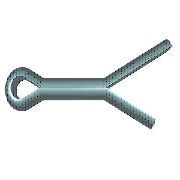
# Autodesk Inventor part: ISO 1234 - 2,5 x 12
Saved by Autodesk Inventor 2024.4 (Build 284460000, 460)
## iProperties
Created: 2023-01-19
Part Number: ISO 1234 - 2,5 x 12
Material: Stahl
Description: Splint
Document SubType Name: Modeling
Standard: ISO 1234
Designer: windows-desktop
Standard Revision: 1998
Standards Organization: DIN
Language: de-DE
Size Designation: 2,5 x 12
Categories: <MemberInstance><Categories><Category DisplayName="Verbindungselemente" InternalName="e4da775c-781d-43d5-af7c-5136215cf5a6" Mnemonic="FSTN"><Category DisplayName="Stifte" InternalName="3b3d1810-ac9b-4ede-8c7f-cc6b956350b0" Mnemonic="PIN"><CategoryParameter DisplayName="Nenndurchmesser" InternalName="6cc331d7-8ea1-4fca-9c9a-55ec966217e5" Mnemonic="nomdia"/><CategoryParameter DisplayName="Nennlänge" InternalName="897bd938-6adf-4e3c-a2d4-0d7cae45eecd" Mnemonic="nomlen"/><Category DisplayName="Splinte" InternalName="4383ab9c-662d-4701-a95a-d5834a9f0a34" Mnemonic="SPLTPIN"><CategoryParameter DisplayName="Bolzendurchmesser" InternalName="761c08f3-f58b-48c9-8a5c-1931069602db" Mnemonic="bltdia"/></Category></Category></Category><Category DisplayName="Datentyp" InternalName="23b78d0f-2648-40c6-8793-ca6db495c9e8" Mnemonic="DATATYPE"><CategoryParameter DisplayName="Anzeigename" InternalName="05415f3d-3907-474b-a020-eb9d644f4cf3" Mnemonic="DISPLAYNAME"/><CategoryParameter DisplayName="Norm" InternalName="0c0a119c-1e12-4c84-803f-101930972f5e" Mnemonic="STANDARD"/><CategoryParameter DisplayName="Beschreibung" InternalName="13903e3d-64b1-4950-80da-f627842ea37f" Mnemonic="DESCRIPTION"/><CategoryParameter DisplayName="Bezeichnung" InternalName="2675968c-4ce5-49e0-a4f5-552d29089031" Mnemonic="DESIGNATION"/><CategoryParameter DisplayName="Standardzeile" InternalName="2af9ec52-faaa-4026-b378-f9fa4afca842" Mnemonic="DEFAULTROW"/><CategoryParameter DisplayName="Ordnername" InternalName="3f06958e-8713-4116-9be7-ed6184ecc97b" Mnemonic="FOLDERNAME"/><CategoryParameter DisplayName="Revisionsanleitung" InternalName="45a75005-10b1-4dfc-8d6d-dfe629f0b93c" Mnemonic="REVISIONGUID"/><CategoryParameter DisplayName="Dateiname" InternalName="8b46a4cc-9585-4fed-90c3-899f57e09a73" Mnemonic="FILENAME"/><CategoryParameter DisplayName="Normungsorganisation" InternalName="8f5914e1-4693-403f-8ab5-d37768198c9d" Mnemonic="STDSORG"/><CategoryParameter DisplayName="Gruppenversion" InternalName="914462f6-6e19-4b14-ba84-155b9680b1d0" Mnemonic="FAMILYREVISION"/><CategoryParameter DisplayName="Normrevision" InternalName="91d5a463-65c2-4fde-b823-3b7fea5e8e17" Mnemonic="STANDARDREVISION"/><CategoryParameter DisplayName="Variantenrevision" InternalName="a65d44b9-392f-4f4f-857b-e4b3d54996fe" Mnemonic="MEMBERREVISION"/><CategoryParameter DisplayName="ClipFormat" InternalName="bc51e27b-3422-4e78-93ef-cec197ddf230" Mnemonic="CLIPFORMAT"/><CategoryParameter DisplayName="Hersteller" InternalName="cd6c7a72-a28a-4e50-99a9-2c7f4e13e5ad" Mnemonic="MANUFACTURER"/><CategoryParameter DisplayName="InternerName" InternalName="cf1d0246-76d9-4b4a-8305-fa0409afb5c1" Mnemonic="INTERNALNAME"/><CategoryParameter DisplayName="IstMetrisch" InternalName="e2385c5b-1ea4-4823-96a8-8de651266ec3" Mnemonic="ISMETRIC"/><Category DisplayName="Bauteil" InternalName="c0e0b642-3bcb-4cc8-9e80-f96d35c4afa4" Mnemonic="PART"><CategoryParameter DisplayName="Bauteilnummer" InternalName="016b6077-bfbe-49bd-92c9-d8d59c39c941" Mnemonic="PARTNUMBER"/><CategoryParameter DisplayName="Bestandsnummer" InternalName="4dba7c1c-e26c-444e-836c-b08b433409a8" Mnemonic="STOCKNUMBER"/><CategoryParameter DisplayName="Materialschlüssel" InternalName="5c9a8adb-dd2b-4535-b97f-0a94a95fe41f" Mnemonic="MATERIALKEY"/><CategoryParameter DisplayName="Material" InternalName="818a152a-d3c3-49ca-80ee-df7d91421b8e" Mnemonic="MATERIAL"/></Category></Category><Category DisplayName="ÄltereVersionenzuweisen" InternalName="cd87c42b-3e48-431e-b5c0-1cbeb14dfe77" Mnemonic="LEGACYMAP"><CategoryParameter DisplayName="Eindeutige DA-Varianten-ID" InternalName="0918ad47-427f-4fed-ae26-24c81c58f590" Mnemonic="DACOOKIE"/><CategoryParameter DisplayName="ID zusammenführen" InternalName="0ee8fb18-e2ed-4f39-96f6-1f4b5f50aa71" Mnemonic="MERGE11"/><CategoryParameter DisplayName="Eindeutige CC-Varianten-ID" InternalName="5193edd4-b2b0-4ab4-9d54-de900eee34e0" Mnemonic="CCCOOKIE"/><CategoryParameter DisplayName="ID aufteilen" InternalName="72b5c83c-be7f-45c4-ae51-9160ea6deb26" Mnemonic="SPLIT"/><CategoryParameter DisplayName="VarianteID" InternalName="8e5e0294-fc51-4c8f-b3d7-003dc5ed94f6" Mnemonic="MEMBERID"/><CategoryParameter DisplayName="Katalogname" InternalName="d99d1e27-aa94-4de2-af4c-c348882a6f4f" Mnemonic="CATALOGNAME"/><CategoryParameter DisplayName="Gruppennummer" InternalName="e705e1f4-09cb-413e-91f9-551b4188271e" Mnemonic="FAMILYNUMBER"/></Category></Categories><FamilyTemplate Id="si0028"><FamilyTemplateParameters><FamilyTemplateParameter ObjectType="kUserParameterObject" ValueType="xs:double" Id="1" ObjectReferenceKey="KBR"/><FamilyTemplateParameter ObjectType="kUserParameterObject" ValueType="xs:double" Id="2" ObjectReferenceKey="NNDMAX"/><FamilyTemplateParameter ObjectType="kUserParameterObject" ValueType="xs:double" Id="3" ObjectReferenceKey="DSH"/><FamilyTemplateParameter ObjectType="kUserParameterObject" ValueType="xs:double" Id="4" ObjectReferenceKey="MSIAB"/><FamilyTemplateParameter ObjectType="kUserParameterObject" ValueType="xs:double" Id="5" ObjectReferenceKey="SNLG"/><FamilyTemplateParameter ObjectType="kUserParameterObject" ValueType="xs:double" Id="6" ObjectReferenceKey="SNND"/><FamilyTemplateParameter ObjectType="kUserParameterObject" ValueType="xs:double" Id="7" ObjectReferenceKey="KOL"/><FamilyTemplateParameter ObjectType="kUserParameterObject" ValueType="xs:double" Id="8" ObjectReferenceKey="LGDIF"/><FamilyTemplateParameter ObjectType="kUserParameterObject" ValueType="xs:double" Id="9" ObjectReferenceKey="NNDMIN"/><FamilyTemplateParameter ObjectType="kUserParameterObject" ValueType="xs:double" Id="10" ObjectReferenceKey="SNND1"/><FamilyTemplateParameter ObjectType="kPropertyObject" ValueType="xs:string" Id="100" ObjectReferenceKey="{32853F0F-3444-11d1-9E93-0060B03C1CA6}" SubObjectId="52"/><FamilyTemplateParameter ObjectType="kPropertyObject" ValueType="xs:string" Id="105" ObjectReferenceKey="{32853F0F-3444-11d1-9E93-0060B03C1CA6}" SubObjectId="5"/><FamilyTemplateParameter ObjectType="kPartComponentDefinitionObject" ValueType="xs:string" Id="110" SubObjectId="Material"/></FamilyTemplateParameters></FamilyTemplate><CategoryParameterMap><ParamToTemplateMap><ParamToTemplate CategoryParameter="//CategoryParameter[@InternalName='05415f3d-3907-474b-a020-eb9d644f4cf3']" ConstantValue="DIN EN ISO 1234"/><ParamToTemplate CategoryParameter="//CategoryParameter[@InternalName='cf1d0246-76d9-4b4a-8305-fa0409afb5c1']" ConstantValue="e94eddc3-8f06-45e0-83a1-c6f48b028452"/><ParamToTemplate CategoryParameter="//CategoryParameter[@InternalName='3f06958e-8713-4116-9be7-ed6184ecc97b']" ConstantValue="ISO 1234(1)"/><ParamToTemplate CategoryParameter="//CategoryParameter[@InternalName='914462f6-6e19-4b14-ba84-155b9680b1d0']" ConstantValue="10"/><ParamToTemplate CategoryParameter="//CategoryParameter[@InternalName='bc51e27b-3422-4e78-93ef-cec197ddf230']" ConstantValue="CF_INVENTOR.STDPARTS"/><ParamToTemplate CategoryParameter="//CategoryParameter[@InternalName='e2385c5b-1ea4-4823-96a8-8de651266ec3']" ConstantValue="true"/><ParamToTemplate CategoryParameter="//CategoryParameter[@InternalName='13903e3d-64b1-4950-80da-f627842ea37f']" ConstantValue="Split Pin"/><ParamToTemplate CategoryParameter="//CategoryParameter[@InternalName='8f5914e1-4693-403f-8ab5-d37768198c9d']" ConstantValue="DIN"/><ParamToTemplate CategoryParameter="//CategoryParameter[@InternalName='0c0a119c-1e12-4c84-803f-101930972f5e']" ConstantValue="ISO 1234"/><ParamToTemplate CategoryParameter="//CategoryParameter[@InternalName='cd6c7a72-a28a-4e50-99a9-2c7f4e13e5ad']" TemplateParameter="104"/><ParamToTemplate CategoryParameter="//CategoryParameter[@InternalName='91d5a463-65c2-4fde-b823-3b7fea5e8e17']" ConstantValue="1998"/><ParamToTemplate CategoryParameter="//CategoryParameter[@InternalName='45a75005-10b1-4dfc-8d6d-dfe629f0b93c']" ConstantValue="dfdbe262-4242-467a-bd84-0a8edc805856"/><ParamToTemplate CategoryParameter="//CategoryParameter[@InternalName='2af9ec52-faaa-4026-b378-f9fa4afca842']" ConstantValue="10"/><ParamToTemplate CategoryParameter="//CategoryParameter[@InternalName='d99d1e27-aa94-4de2-af4c-c348882a6f4f']" ConstantValue="DIN"/><ParamToTemplate CategoryParameter="//CategoryParameter[@InternalName='e705e1f4-09cb-413e-91f9-551b4188271e']" ConstantValue="220"/><ParamToTemplate CategoryParameter="//CategoryParameter[@InternalName='8b46a4cc-9585-4fed-90c3-899f57e09a73']" ConstantValue="ISO 1234 - 2,5 x 12DIN EN"/><ParamToTemplate CategoryParameter="//CategoryParameter[@InternalName='a65d44b9-392f-4f4f-857b-e4b3d54996fe']" ConstantValue="35897454-1E07-4AEE-A925-0F5C18AD98F7"/><ParamToTemplate CategoryParameter="//CategoryParameter[@InternalName='8e5e0294-fc51-4c8f-b3d7-003dc5ed94f6']" ConstantValue="540"/><ParamToTemplate CategoryParameter="//CategoryParameter[@InternalName='2675968c-4ce5-49e0-a4f5-552d29089031']" TemplateParameter="100"/><ParamToTemplate CategoryParameter="//CategoryParameter[@InternalName='818a152a-d3c3-49ca-80ee-df7d91421b8e']" TemplateParameter="110"/><ParamToTemplate CategoryParameter="//CategoryParameter[@InternalName='761c08f3-f58b-48c9-8a5c-1931069602db']" TemplateParameter="2"/><ParamToTemplate CategoryParameter="//CategoryParameter[@InternalName='016b6077-bfbe-49bd-92c9-d8d59c39c941']" TemplateParameter="105"/><ParamToTemplate CategoryParameter="//CategoryParameter[@InternalName='897bd938-6adf-4e3c-a2d4-0d7cae45eecd']" TemplateParameter="5"/><ParamToTemplate CategoryParameter="//CategoryParameter[@InternalName='6cc331d7-8ea1-4fca-9c9a-55ec966217e5']" TemplateParameter="6"/></ParamToTemplateMap></CategoryParameterMap></MemberInstance>
Mass: 0.700909 g
Surface Area: 2.16494 cm^2
Volume: 0.0892877 cm^3
Density: 7.85 g/cm^3
Appearance: Platte
IsCustomPart: 0
Author: windows-desktop
Autodesk Inventor part; units mm, degrees
ref_plane "YZ Plane" through (0, 0, 0) normal (1, 0, 0) x (0, 1, 0)
sketch "Skizze1" plane through (0, 0, 0) normal (0, 1, 0) x (-1, 0, 0)
  arc A0 (-1.6014, 2.0207) -> (-1.6014, -2.0207) centre (-2.7, 0) ccw
  arc A1 (-2.2102, 1.0405) -> (-2.2102, -1.0405) centre (-2.7, 0) ccw
  line L0 (0, 1.15) -> (6, 1.15)
  line L1 (0, -1.15) -> (6, -1.15)
  line L2 (6, 1.15) -> (12, 3.4487)
  line L3 (12, 3.4487) -> (12.3842, 2.4459)
  line L4 (12.3842, 2.4459) -> (6, 0)
  line L5 (6, 0) -> (14.8842, -3.4037)
  line L6 (14.8842, -3.4037) -> (14.5, -4.4065)
  line L7 (14.5, -4.4065) -> (6, -1.15)
  line L8 (0, 0) -> (-2.2102, -1.0405)
  line L9 (0, 0) -> (-2.2102, 1.0405)
  line L10 (0, 1.15) -> (0, -1.15) construction
  line L11 (0, 1.15) -> (-1.6014, 2.0207)
  line L12 (0, -1.15) -> (-1.6014, -2.0207)
  line L13 (-5, 0) -> (6, 0) construction
  line L14 (6, 1.15) -> (6, -1.15) construction
  dimension "d0" = 6
  dimension "d1" = 12
  dimension "d2" = 159.037
  dimension "d3" = 159.037
  dimension "d4" = 2.5
  dimension "d5" = 1.15
  dimension "d6" = 2.3
  dimension "d7" = 1.15
  dimension "d8" = 1.15
  dimension "d9" = 2.7
  constraints: 30 end point, 5 point on circle, 4 parallel, 4 perpendicular, 4 point on line, 4 tangent, 2 centre point, 2 midpoint, 1 coincident, 1 horizontal
  measures "d0" distance of L0.start L0.end
  measures "d1" horizontal distance of L0.start L2.end
  measures "d2" angle of L0 L2
  measures "d3" angle of L1 L7
  measures "d4" horizontal distance of L2.end L6.end
  measures "d5" radius of A1
  measures "d6" radius of A0
  measures "d7" distance from line of L0 L8.start
  measures "d8" distance between parallel lines of L1 L13
  measures "d9" distance from line of L10 A0.centre
extrude "Körper" add sketch "Skizze1" along normal mid plane 2.3
fillet "Rundung" radius 0.805 14 edges at (-9, -1.15, 2.2994) (-9, 1.15, 2.2994) (-3, -1.15, 1.15) (-3, 1.15, 1.15) (5, -1.15, 0) (0.8007, -1.15, -1.5853) (0.8007, -1.15, 1.5853) (5, 1.15, 0) (0.8007, 1.15, 1.5853) (0.8007, 1.15, -1.5853) (-3, -1.15, -1.15) (-10.25, -1.15, -2.7783) (-3, 1.15, -1.15) (-10.25, 1.15, -2.7783)
ref_plane "Work Plane1" through (0, -10, 0) normal (0, 0, -1) x (0, 1, 0)
ref_plane "Work Plane3" through (0, 0, 1.15) normal (-1, 0, 0) x (0, 1, 0)
equation "\"d0\" = MSIAB"
equation "\"d1\" = SNLG"
equation "\"d4\" = LGDIF"
equation "\"d5\" = -0.5 * SNND1 + 0.5 * KBR"
equation "\"d6\" = 0.5 * KBR"
equation "\"d7\" = 0.5 * SNND1"
equation "\"d8\" = 0.5 * SNND1"
equation "\"d9\" = KOL - 0.5 * KBR"
equation "\"d10\" = SNND1"
equation "\"d12\" = 0.35 * SNND1"
equation "\"SNND\" = 2.5"
equation "\"SNLG\" = 12"
equation "\"SNND1\" = 2.3"
equation "\"KBR\" = 4.6"
equation "\"KOL\" = 5"
equation "\"LGDIF\" = 2.5"
equation "\"MSIAB\" = 6"
equation "\"NNDMAX\" = 11"
equation "\"DSH\" = 5"
equation "\"NNDMIN\" = 9"
body "Solid1"
